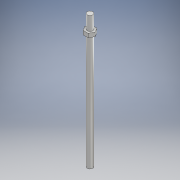
# Autodesk Inventor part: aircylinder16_100_part2_sa
Saved by Autodesk Inventor 2018 (Build 220112000, 112)
## iProperties
Created: 2018-03-06
Part Number: aircylinder16_100_part2_sa
Material: アルミニウム 6061-AHC
Document SubType Name: Modeling
Designer: shun
Density: 2.7 g/cm^3
Appearance: アルミニウム - ダーク
Author: shun
Autodesk Inventor part; units mm, degrees
ref_plane "YZ Plane" through (0, 0, 0) normal (1, 0, 0) x (0, 1, 0)
ref_plane "XZ Plane" through (0, 0, 0) normal (0, 1, 0) x (-1, 0, 0)
ref_plane "XY Plane" through (0, 0, 0) normal (0, 0, 1) x (1, 0, 0)
sketch "スケッチ1" plane through (0, 0, 0) normal (0, 0, 1) x (1, 0, 0)
  circle A0 centre (0, 0) radius 2.5
  dimension "d0" = 5
  constraints: 1 centre point, 1 coincident
  measures "d0" diameter of A0
extrude "押し出し1" add sketch "スケッチ1" along normal blind 104
sketch "スケッチ2" plane through (0, 0, 104) normal (0, 0, 1) x (1, 0, 0)
  line L0 (4.6188, 0) -> (2.3094, -4)
  line L1 (2.3094, -4) -> (-2.3094, -4)
  line L2 (-2.3094, -4) -> (-4.6188, 0)
  line L3 (-4.6188, 0) -> (-2.3094, 4)
  line L4 (-2.3094, 4) -> (2.3094, 4)
  line L5 (2.3094, 4) -> (4.6188, 0)
  point P0 (0, 0)
  point P1 (0, 0)
  dimension "d3" = 8
  constraints: 12 end point, 1 coincident, 13 other
  measures "d3" distance between parallel lines of L1 L4
extrude "押し出し2" add sketch "スケッチ2" along normal blind 3.5
sketch "スケッチ3" plane through (0, 0, 107.5) normal (0, 0, 1) x (1, 0, 0)
  circle A0 centre (0, 0) radius 2.5
  dimension "d6" = 5
  constraints: 1 centre point, 1 coincident
  measures "d6" diameter of A0
extrude "押し出し3" add sketch "スケッチ3" along normal blind 12.5
